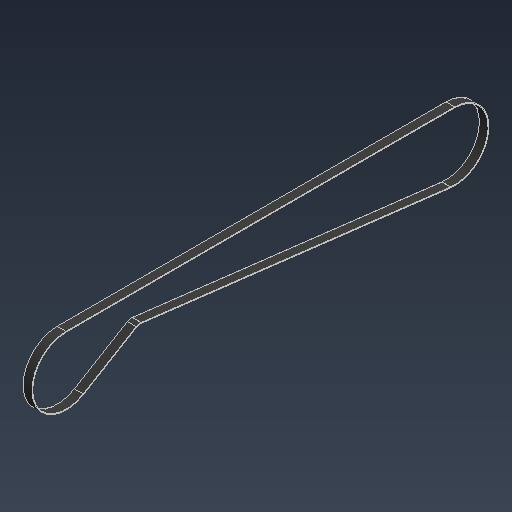
# Autodesk Inventor part: belt_1
Saved by Autodesk Inventor 2021 (Build 250183000, 183)
## iProperties
Created: 2021-07-18
Part Number: belt_1
Material: ゴム
Document SubType Name: Modeling
Designer: yuta0
Density: 0.93 g/cm^3
Appearance: ゴム - 黒
Mass: 8.55769 g
Surface Area: 248.449 cm^2
Volume: 9.20182 cm^3
購入先: ミスミ
在庫数: 0.0
Author: yuta0
Autodesk Inventor part; units mm, degrees
ref_plane "YZ Plane" through (0, 0, 0) normal (1, 0, 0) x (0, 1, 0)
ref_plane "XZ Plane" through (0, 0, 0) normal (0, 1, 0) x (-1, 0, 0)
ref_plane "XY Plane" through (0, 0, 0) normal (0, 0, 1) x (1, 0, 0)
sketch "スケッチ1" plane through (0, 0, 0) normal (1, 0, 0) x (0, 1, 0)
  arc A0 (38.1972, 0) -> (-32.7626, -19.6376) centre (0, 0) ccw
  arc A1 (-37.9221, -435.4244) -> (38.1972, -440) centre (0, -440) ccw
  arc A2 (4.3584, -85.0085) -> (3.2212, -79.6717) centre (-4, -84) ccw
  line L0 (3.2212, -79.6717) -> (-32.7626, -19.6376)
  line L1 (38.1972, -440) -> (38.1972, 0)
  line L2 (4.3584, -85.0085) -> (-37.9221, -435.4244)
  arc A3 (38.6162, 0) -> (-33.122, -19.853) centre (0, 0) ccw
  line L3 (-33.122, -19.853) -> (2.8618, -79.8871)
  arc A4 (3.9424, -84.9583) -> (2.8618, -79.8871) centre (-4, -84) ccw
  line L4 (3.9424, -84.9583) -> (-38.3381, -435.3742)
  arc A5 (-38.3381, -435.3742) -> (38.6162, -440) centre (0, -440) ccw
  line L5 (38.6162, -440) -> (38.6162, 0)
  arc A6 (37.8162, 0) -> (-32.4358, -19.4417) centre (0, 0) ccw
  line L6 (-32.4358, -19.4417) -> (3.548, -79.4758)
  arc A7 (4.7366, -85.0541) -> (3.548, -79.4758) centre (-4, -84) ccw
  line L7 (4.7366, -85.0541) -> (-37.5439, -435.47)
  arc A8 (-37.5439, -435.47) -> (37.8162, -440) centre (0, -440) ccw
  line L8 (37.8162, -440) -> (37.8162, 0)
  dimension "d0" = 76.3944
  dimension "d1" = 76.3944
  dimension "d2" = 440
  dimension "d24" = 0.419
  dimension "d25" = 8
  dimension "d26" = 84
  dimension "d27" = 0.8
  dimension "d30" = 4
  constraints: 18 end point, 18 point on circle, 9 centre point, 6 tangent, 1 coincident, 1 vertical alignment, 10 other
  measures "d0" diameter of A0
  measures "d1" diameter of A1
  measures "d2" distance of A0.centre A1.centre
  measures "d24" distance between parallel lines of L1 L5
  measures "d25" radius of A4
  measures "d26" vertical distance of point (0, 0) A2.centre
  measures "d27" distance between parallel lines of L5 L8
  measures "d30" horizontal distance of point (0, 0) A2.centre
extrude "押し出し1" add sketch "スケッチ1" along normal mid plane 10 contours L1 A1 L2 A2 L0 A0 | L5 A5 L4 A4 L3 A3
